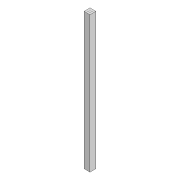
# Autodesk Inventor part: post-tall
Saved by Autodesk Inventor 2020 (Build 240168000, 168)
## iProperties
Created: 2021-06-08
Part Number: post-tall
Material: Generic
Document SubType Name: Modeling
Designer: Aidan Lee
Density: 1 g/cm^3
Appearance: Default
Author: Aidan Lee
Autodesk Inventor part; units mm, degrees
ref_plane "YZ Plane" through (0, 0, 0) normal (1, 0, 0) x (0, 1, 0)
ref_plane "XZ Plane" through (0, 0, 0) normal (0, 1, 0) x (-1, 0, 0)
ref_plane "XY Plane" through (0, 0, 0) normal (0, 0, 1) x (1, 0, 0)
sketch "Sketch1" plane through (0, 0, 0) normal (0, 1, 0) x (-1, 0, 0)
  line L0 (69, 69) -> (0, 69)
  line L1 (0, 69) -> (0, 0)
  line L2 (0, 0) -> (69, 0)
  line L3 (69, 0) -> (69, 69)
  dimension "d0" = 69
  dimension "d1" = 69
  constraints: 8 end point, 2 parallel, 1 coincident, 1 horizontal, 1 perpendicular
  measures "d0" distance of L1.end L2.end
  measures "d1" distance of L0.end L1.end
extrude "Extrusion1" add sketch "Sketch1" along normal blind 1582
sketch "Sketch2" plane through (0, 1582, 0) normal (0, 1, 0) x (1, 0, 0)
  circle A0 centre (-46, -46) radius 2.5
  circle A1 centre (-23, -23) radius 2.5
  circle A2 centre (-46, -23) radius 2.5
  circle A3 centre (-23, -46) radius 2.5
  line L0 (0, 0) -> (-69, 0) projected
  line L1 (0, -69) -> (0, 0) projected
  line L2 (-23, -23) -> (-46, -46)
  line L3 (-46, -23) -> (-23, -46)
  line L4 (-69, 0) -> (-69, -69) projected
  point P0 (-34.5, -34.5)
  point P1 (0, -34.5)
  point P2 (-34.5, 0)
  dimension "screwhole" = 5
  dimension "d23" = 5
  dimension "d24" = 5
  dimension "d25" = 5
  dimension "d26" = 23
  constraints: 4 centre point, 4 end point, 3 horizontal alignment, 3 midpoint, 3 vertical alignment, 1 perpendicular
  measures "screwhole" diameter of A0
  measures "d23" diameter of A3
  measures "d24" diameter of A1
  measures "d25" diameter of A2
  measures "d26" distance from line of L4 L2.end
extrude "Extrusion2" cut sketch "Sketch2" against normal blind 85
equation "\"d23\" = screwhole"
equation "\"d24\" = screwhole"
equation "\"d25\" = screwhole"
body "Solid1"
